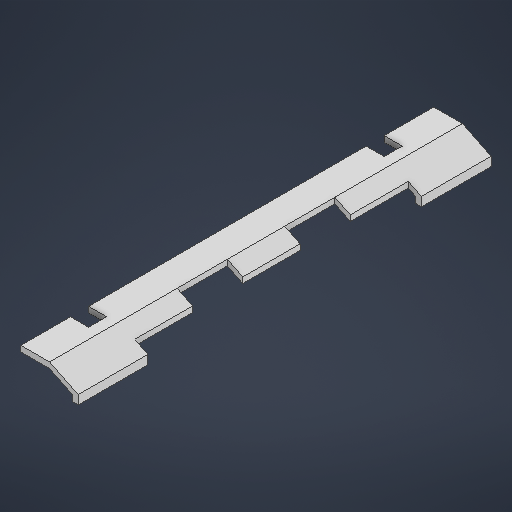
# Autodesk Inventor part: prrzod
Saved by Autodesk Inventor 2026.2 (Build 302298010, 298A)
## iProperties
Created: 2026-05-09
Part Number: prrzod
Material: Ogólny
Document SubType Name: Modeling
Designer: karol
Density: 1 g/cm^3
Appearance: Domyślna
Author: karol
Autodesk Inventor part; units mm, degrees
ref_plane "YZ Plane" through (0, 0, 0) normal (1, 0, 0) x (0, 1, 0)
ref_plane "XZ Plane" through (0, 0, 0) normal (0, 1, 0) x (-1, 0, 0)
ref_plane "XY Plane" through (0, 0, 0) normal (0, 0, 1) x (1, 0, 0)
sketch "Szkic32" plane through (0, 0, 0) normal (0, 0, 1) x (1, 0, 0)
  line L0 (0, 0) -> (10, 0)
  line L1 (10, 0) -> (15.9865, -2.9108)
  line L2 (10, 0) -> (16.6566, 0) construction
  line L3 (10, 0) -> (20.0005, -4.8625)
  line L4 (20.0005, -4.8625) -> (20.0005, -7.9995)
  line L5 (20.0005, -7.9995) -> (18.0005, -7.9995)
  line L6 (0, 0) -> (0, -2)
  line L7 (0, -2) -> (10, -2)
  line L8 (10, -2) -> (18.0005, -5.89)
  line L9 (10, -2) -> (18.8961, -2) construction
  line L10 (18.0005, -5.89) -> (18.0005, -7.9995)
  dimension "d102" = 10
  dimension "d103" = 25.93
  dimension "d104" = 11.12
  dimension "d105" = 3.137
  dimension "d106" = 2
  dimension "d107" = 2
  dimension "d108" = 10
  dimension "d109" = 25.93
  constraints: 22 end point, 3 horizontal, 3 vertical, 2 equal length, 2 perpendicular, 1 point on line
  measures "d102" distance of L0.start L0.end
  measures "d103" angle of L1 L2
  measures "d104" distance of L0.end L3.end
  measures "d105" distance of L3.end L4.end
  measures "d106" distance of L4.end L5.end
  measures "d107" distance of L0.start L6.end
  measures "d108" distance of L6.end L7.end
  measures "d109" angle of L8 L9
extrude "Wyciągnięcie proste35" add sketch "Szkic32" along normal blind 24.3
sketch "Szkic33" plane through (0, 0, 24.3) normal (0, 0, 1) x (1, 0, 0)
  line L0 (10, 0) -> (0, 0) projected
  line L1 (0, 0) -> (0, -2) projected
  line L2 (0, -2) -> (10, -2) projected
  line L3 (0, 0) -> (10, 0)
  line L4 (10, 0) -> (10, -2)
  line L5 (10, -2) -> (0, -2)
  line L6 (0, -2) -> (0, 0)
  line L7 (10, -2) -> (15.396, -4.6236)
  line L8 (10, -2) -> (18.0005, -5.89) projected
  line L9 (15.396, -4.6236) -> (15.396, -2.6236)
  line L10 (20.0005, -4.8625) -> (10, 0) projected
  line L11 (10, 0) -> (15.396, -2.6236)
  dimension "d112" = 6
  constraints: 14 end point, 3 parallel, 2 point on line, 1 horizontal, 1 perpendicular, 1 vertical
  measures "d112" distance of L2.end L7.end
extrude "Wyciągnięcie proste36" add sketch "Szkic33" along normal blind 20.2
sketch "Szkic34" plane through (0, 0, 44.5) normal (0, 0, 1) x (1, 0, 0)
  line L0 (10, 0) -> (0, 0) projected
  line L1 (0, -2) -> (10, -2) projected
  line L2 (0, 0) -> (10, 0)
  line L3 (10, 0) -> (10, -2)
  line L4 (10, -2) -> (0, -2)
  line L5 (0, -2) -> (0, 0)
  constraints: 8 end point, 2 parallel, 1 horizontal, 1 perpendicular
extrude "Wyciągnięcie proste37" add sketch "Szkic34" along normal blind 17.5
sketch "Szkic36" plane through (0, 0, 62) normal (0, 0, 1) x (1, 0, 0)
  line L0 (15.396, -2.6236) -> (10, 0) projected
  line L1 (15.396, -4.6236) -> (15.396, -2.6236) projected
  line L2 (10, -2) -> (15.396, -4.6236) projected
  line L3 (0, -2) -> (10, -2) projected
  line L4 (10, 0) -> (0, 0) projected
  line L5 (0, 0) -> (0, -2) projected
  line L6 (10, 0) -> (15.396, -2.6236)
  line L7 (15.396, -2.6236) -> (15.396, -4.6236)
  constraints: 4 end point, 2 collinear
extrude "Wyciągnięcie proste38" add sketch "Szkic36" along normal blind 20
sketch "Szkic37" plane through (0, 0, 82) normal (0, 0, 1) x (1, 0, 0)
  line L0 (10, 0) -> (0, 0) projected
  line L1 (0, -2) -> (10, -2) projected
  line L2 (0, 0) -> (10, 0)
  line L3 (10, 0) -> (10, -2)
  line L4 (10, -2) -> (0, -2)
  line L5 (0, -2) -> (0, 0)
  constraints: 8 end point, 2 parallel, 1 horizontal, 1 perpendicular
extrude "Wyciągnięcie proste39" add sketch "Szkic37" along normal blind 17.5
sketch "Szkic38" plane through (0, 0, 99.5) normal (0, 0, 1) x (1, 0, 0)
  line L0 (15.396, -2.6236) -> (10, 0) projected
  line L1 (15.396, -4.6236) -> (15.396, -2.6236) projected
  line L2 (10, -2) -> (15.396, -4.6236) projected
  line L3 (0, -2) -> (10, -2) projected
  line L4 (10, 0) -> (0, 0) projected
  line L5 (10, 0) -> (0, 0) projected
  line L6 (0, 0) -> (0, -2) projected
  line L7 (0, -2) -> (10, -2) projected
  line L8 (10, -2) -> (10, 0) projected
extrude "Wyciągnięcie proste40" add sketch "Szkic38" along normal blind 20.2
sketch "Szkic39" plane through (0, 0, 119.7) normal (0, 0, 1) x (1, 0, 0)
  line L0 (15.396, -2.6236) -> (15.396, -4.6236) projected
  line L1 (15.396, -4.6236) -> (18.0005, -5.89) projected
  line L2 (18.0005, -5.89) -> (18.0005, -7.9995) projected
  line L3 (18.0005, -7.9995) -> (20.0005, -7.9995) projected
  line L4 (20.0005, -7.9995) -> (20.0005, -4.8625) projected
  line L5 (20.0005, -4.8625) -> (15.396, -2.6236) projected
  line L6 (0, 0) -> (0, -2) projected
  line L7 (0, -2) -> (10, -2) projected
  line L8 (10, -2) -> (15.396, -4.6236) projected
  line L9 (15.396, -4.6236) -> (15.396, -2.6236) projected
  line L10 (15.396, -2.6236) -> (10, 0) projected
  line L11 (10, 0) -> (0, 0) projected
extrude "Wyciągnięcie proste41" add sketch "Szkic39" along normal blind 24.3
sketch "Szkic40" plane through (0, 0, 0) normal (0, 1, 0) x (1, 0, 0)
  line L0 (0, 0) -> (0, -144) projected
  line L1 (0, -17.3) -> (6.3, -17.3)
  line L2 (6.3, -17.3) -> (6.3, -23.6)
  line L3 (6.3, -23.6) -> (0, -23.6)
  line L4 (0, -23.6) -> (0, -17.3)
  line L5 (10, 0) -> (0, 0) projected
  line L6 (0, -126.7) -> (6.3, -126.7)
  line L7 (6.3, -126.7) -> (6.3, -120.4)
  line L8 (6.3, -120.4) -> (0, -120.4)
  line L9 (0, -120.4) -> (0, -126.7)
  line L10 (10, -144) -> (0, -144) projected
  point P0 (0, -120.4)
  point P1 (0, -23.6)
  dimension "d125" = 6.3
  dimension "d126" = 6.3
  dimension "d127" = 17.3
  dimension "d128" = 6.3
  dimension "d129" = 6.3
  dimension "d130" = 17.3
  constraints: 16 end point, 4 parallel, 2 horizontal, 2 perpendicular, 2 point on line
  measures "d125" distance of L2.end L3.end
  measures "d126" distance of L1.end L2.end
  measures "d127" distance between parallel lines of L5 L1
  measures "d128" distance of L8.end L7.end
  measures "d129" distance of L7.end L6.end
  measures "d130" distance between parallel lines of L10 L6
extrude "Wyciągnięcie proste42" cut sketch "Szkic40" against normal blind 2
